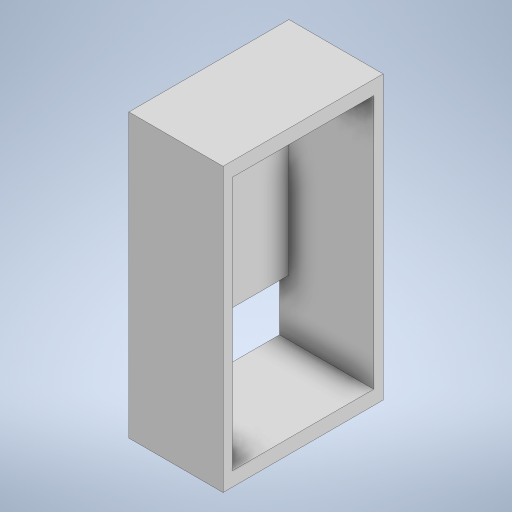
# Autodesk Inventor part: support_tof_actionneur_panneaux_solaires
Saved by Autodesk Inventor 2024.1 (Build 281209000, 209)
## iProperties
Created: 2024-04-13
Part Number: support_tof_actionneur_panneaux_solaires
Material: Générique
Document SubType Name: Modeling
Designer: chass
Density: 1 g/cm^3
Appearance: Par défaut
Author: chass
Autodesk Inventor part; units mm, degrees
ref_plane "YZ Plane" through (0, 0, 0) normal (1, 0, 0) x (0, 1, 0)
ref_plane "XZ Plane" through (0, 0, 0) normal (0, 1, 0) x (-1, 0, 0)
ref_plane "XY Plane" through (0, 0, 0) normal (0, 0, 1) x (1, 0, 0)
sketch "Esquisse1" plane through (0, 0, 0) normal (1, 0, 0) x (0, 1, 0)
  line L0 (15, 8.5) -> (-15, 8.5)
  line L1 (-15, 8.5) -> (-15, -8.5)
  line L2 (-15, -8.5) -> (15, -8.5)
  line L3 (15, -8.5) -> (15, 8.5)
  point P0 (0, 0)
  point P1 (0, 0)
  point P2 (0, 0)
  dimension "d4" = 30
  dimension "d5" = 17
  constraints: 8 end point, 2 parallel, 1 coincident, 1 horizontal, 1 perpendicular
  measures "d4" distance of L1.end L2.end
  measures "d5" distance of L2.end L0.start
extrude "Extrusion1" add sketch "Esquisse1" along normal blind 10
sketch "Esquisse2" plane through (10, 0, 0) normal (1, 0, 0) x (0, 0, -1)
  line L0 (-7.5, 13.5) -> (7.5, 13.5)
  line L1 (7.5, 13.5) -> (7.5, -13.5)
  line L2 (7.5, -13.5) -> (-7.5, -13.5)
  line L3 (-7.5, -13.5) -> (-7.5, 13.5)
  line L4 (-7.5, 13.5) -> (7.5, -13.5)
  line L5 (-7.5, -13.5) -> (7.5, 13.5)
  point P0 (0, 0)
  point P1 (0, 0)
  point P2 (0, 0)
  dimension "d8" = 27
  dimension "d9" = 15
  constraints: 12 end point, 2 midpoint, 2 parallel, 1 coincident, 1 horizontal, 1 perpendicular
  measures "d8" distance of L0.end L1.end
  measures "d9" distance of L0.start L0.end
extrude "Extrusion2" cut sketch "Esquisse2" against normal blind 9
sketch "Esquisse3" plane through (1, 0, 0) normal (1, 0, 0) x (0, 0, -1)
  line L0 (7.5, -13.5) -> (-7.5, -13.5) projected
  line L1 (7.5, 13.5) -> (7.5, -13.5) projected
  line L2 (-7.5, -13.5) -> (7.5, -13.5)
  line L3 (7.5, -13.5) -> (7.5, -7.5)
  line L4 (7.5, -7.5) -> (-7.5, -7.5)
  line L5 (-7.5, -7.5) -> (-7.5, -13.5)
  point P0 (0, 0)
  dimension "d12" = 6
  constraints: 8 end point, 2 parallel, 1 horizontal, 1 perpendicular, 1 point on line
  measures "d12" distance of L3.end L2.end
extrude "Extrusion3" cut sketch "Esquisse3" against normal blind 9
